# Autodesk Inventor part: CHIPLED_0603
Saved by Autodesk Inventor 2016 SP1 (Build 200210100, 210)
## iProperties
Created: 2015-11-24
Part Number: CHIPLED_0603
Material: Generic
Document SubType Name: Modeling
Designer: PhillipD
Density: 1 g/cm^3
Appearance: CHIPLED_0603, CHIPLED_0603
Author: PhillipD
Autodesk Inventor part; units mm, degrees
ref_plane "YZ Plane" through (0, 0, 0) normal (1, 0, 0) x (0, 1, 0)
ref_plane "XZ Plane" through (0, 0, 0) normal (0, 1, 0) x (-1, 0, 0)
ref_plane "XY Plane" through (0, 0, 0) normal (0, 0, 1) x (1, 0, 0)
sketch "CHIPLED_0603, CHIPLED_0603_83" plane through (0, 0, 0) normal (0, 0, 1) x (1, 0, 0)
  line L0 (-0.4504, 0.8508) -> (0.45, 0.8508)
  line L1 (0.45, 0.8508) -> (0.45, -0.85)
  line L2 (0.45, -0.85) -> (-0.4504, -0.85)
  line L3 (-0.4504, -0.85) -> (-0.4504, 0.8508)
  constraints: 8 end point
extrude "Extrusion1" add sketch "CHIPLED_0603, CHIPLED_0603_83" along normal blind 1
body "Solid1"
